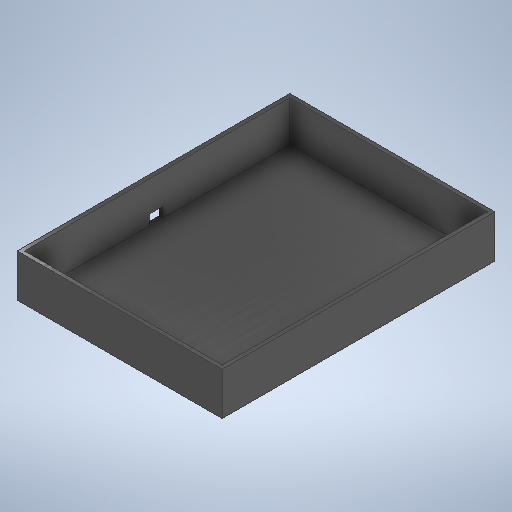
# Autodesk Inventor part: BaseFloor
Saved by Autodesk Inventor 2026.2 (Build 302298010, 298A)
## iProperties
Created: 2026-03-17
Part Number: BaseFloor
Material: Ogólny
Document SubType Name: Modeling
Designer: Patryk
Density: 1 g/cm^3
Appearance: Domyślna
Author: Patryk
Autodesk Inventor part; units mm, degrees
ref_plane "YZ Plane" through (0, 0, 0) normal (1, 0, 0) x (0, 1, 0)
ref_plane "XZ Plane" through (0, 0, 0) normal (0, 1, 0) x (-1, 0, 0)
ref_plane "XY Plane" through (0, 0, 0) normal (0, 0, 1) x (1, 0, 0)
sketch "Szkic1" plane through (0, 0, 0) normal (0, 1, 0) x (-1, 0, 0)
  line L0 (-151.5, -201.5) -> (151.5, -201.5)
  line L1 (151.5, -201.5) -> (151.5, 201.5)
  line L2 (151.5, 201.5) -> (-151.5, 201.5)
  line L3 (-151.5, 201.5) -> (-151.5, -201.5)
  line L4 (-151.5, -201.5) -> (151.5, 201.5) construction
  line L5 (151.5, -201.5) -> (-151.5, 201.5) construction
  point P0 (0, 0)
  dimension "d0" = 403
  dimension "d1" = 303
  constraints: 12 end point, 2 midpoint, 2 parallel, 1 horizontal, 1 perpendicular
  measures "d0" distance of L2.end L0.start
  measures "d1" distance of L1.end L2.end
extrude "Wyciągnięcie proste1" add sketch "Szkic1" along normal mid plane 3
sketch "Szkic2" plane through (0, 1.5, 0) normal (0, 1, 0) x (1, 0, 0)
  line L0 (146, -196) -> (-146, -196)
  line L1 (-146, -196) -> (-146, 196)
  line L2 (-146, 196) -> (146, 196)
  line L3 (146, 196) -> (146, -196)
  line L4 (146, -196) -> (-146, 196) construction
  line L5 (-146, -196) -> (146, 196) construction
  line L6 (-151.5, 201.5) -> (-151.5, -201.5) projected
  line L7 (-151.5, -201.5) -> (151.5, -201.5) projected
  line L8 (151.5, -201.5) -> (151.5, 201.5) projected
  line L9 (151.5, 201.5) -> (-151.5, 201.5) projected
  point P0 (0, 0)
  dimension "d4" = 292
  dimension "d5" = 392
  constraints: 12 end point, 2 midpoint, 2 parallel, 1 horizontal, 1 perpendicular
  measures "d4" distance between parallel lines of L3 L1
  measures "d5" distance between parallel lines of L0 L2
extrude "Wyciągnięcie proste2" add sketch "Szkic2" along normal blind 60
sketch "Szkic4" plane through (-151.5, -1.5, -201.5) normal (-1, 0, 0) x (0, 0, 1)
  line L0 (397.5, 3) -> (5.5, 3) projected
  line L1 (193, 3) -> (213, 3)
  line L2 (213, 3) -> (213, 18)
  line L3 (213, 18) -> (193, 18)
  line L4 (193, 18) -> (193, 3)
  line L5 (403, 0) -> (403, 63) projected
  point P0 (201.5, 1.5)
  dimension "d13" = 20
  dimension "d14" = 15
  dimension "d15" = 190
  constraints: 8 end point, 2 parallel, 1 horizontal, 1 perpendicular, 1 point on line
  measures "d13" distance of L2.end L3.end
  measures "d14" distance of L3.end L1.start
  measures "d15" distance between parallel lines of L5 L2
extrude "Wyciągnięcie proste4" cut sketch "Szkic4" against normal up to surface (5.5 mm away)
